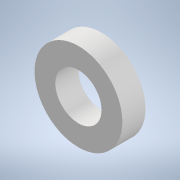
# Autodesk Inventor part: Part6
Saved by Autodesk Inventor 2020.2 (Build 242310000, 310)
## iProperties
Created: 2022-11-14
Part Number: Part6
Material: 一般
Document SubType Name: Modeling
Designer: Administrator
Density: 1 g/cm^3
Appearance: 既定
Author: Administrator
Autodesk Inventor part; units mm, degrees
ref_plane "YZ Plane" through (0, 0, 0) normal (1, 0, 0) x (0, 1, 0)
ref_plane "XZ Plane" through (0, 0, 0) normal (0, 1, 0) x (-1, 0, 0)
ref_plane "XY Plane" through (0, 0, 0) normal (0, 0, 1) x (1, 0, 0)
sketch "スケッチ1" plane through (0, 0, 0) normal (0, 0, 1) x (1, 0, 0)
  circle A0 centre (-13.1683, -17.7882) radius 5 projected
  circle A1 centre (-13.1683, -17.7882) radius 5
  circle A2 centre (-13.1683, -17.7882) radius 9.5
  point P0 (0, 0)
  dimension "d0" = 19
  constraints: 2 centre point, 2 coincident, 1 concentric
  measures "d0" diameter of A2
extrude "押し出し1" add sketch "スケッチ1" along normal blind 5
